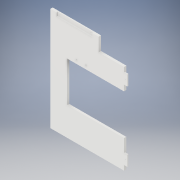
# Autodesk Inventor part: TC001b
Saved by Autodesk Inventor 2017 SP1 (Build 210196100, 196)
## iProperties
Created: 2018-01-07
Part Number: TC001b
Material: ABS Plastic
Document SubType Name: Modeling
Designer: Zach
Density: 1.06 g/cm^3
Appearance: CR White
Author: Zach
Autodesk Inventor part; units mm, degrees
ref_plane "YZ Plane" through (0, 0, 0) normal (1, 0, 0) x (0, 1, 0)
ref_plane "XZ Plane" through (0, 0, 0) normal (0, 1, 0) x (-1, 0, 0)
ref_plane "XY Plane" through (0, 0, 0) normal (0, 0, 1) x (1, 0, 0)
sketch "Sketch1" plane through (0, 0, 0) normal (0, 0, 1) x (1, 0, 0)
  line L0 (0, 0) -> (620, 0)
  line L1 (620, 0) -> (620, 620)
  line L2 (620, 620) -> (0, 620)
  line L3 (0, 620) -> (0, 0)
  line L4 (203.5, 491) -> (416.5, 491)
  line L5 (416.5, 491) -> (416.5, 378)
  line L6 (416.5, 378) -> (203.5, 378)
  line L7 (203.5, 378) -> (203.5, 491)
  point P0 (310, 491)
  point P1 (310, 620)
  dimension "d0" = 620
  dimension "d1" = 620
  dimension "d2" = 213
  dimension "d3" = 113
  dimension "d4" = 129
  constraints: 16 end point, 4 parallel, 2 horizontal, 2 midpoint, 2 perpendicular, 1 vertical alignment
  measures "d0" distance of L2.end L1.end
  measures "d1" distance of L1.end L0.end
  measures "d2" distance of L5.end L6.end
  measures "d3" distance of L4.end L5.end
  measures "d4" distance between parallel lines of L2 L4
extrude "Extrusion1" add sketch "Sketch1" along normal blind 10
sketch "Sketch2" plane through (0, 0, 10) normal (0, 0, 1) x (1, 0, 0)
  line L0 (0, 0) -> (310, 0)
  line L1 (310, 0) -> (310, 435)
  line L2 (310, 435) -> (0, 435)
  line L3 (0, 435) -> (0, 0)
  line L4 (620, 620) -> (0, 620) projected
  line L5 (0, 435) -> (620, 435)
  line L6 (620, 435) -> (620, 620)
  line L7 (620, 620) -> (0, 620)
  line L8 (0, 620) -> (0, 435)
  line L9 (310, 435) -> (620, 435)
  line L10 (620, 435) -> (620, 0)
  line L11 (620, 0) -> (310, 0)
  line L12 (310, 0) -> (310, 435)
  point P0 (310, 620)
  dimension "d7" = 435
  constraints: 24 end point, 6 parallel, 3 horizontal, 3 perpendicular, 1 midpoint, 1 vertical alignment
  measures "d7" distance of L1.end L0.end
extrude "Extrusion2" cut sketch "Sketch2" against normal through all contours L1 L5 L10 L11 | L8 L4 L6 L5 L2
sketch "Sketch3" plane through (0, 0, 10) normal (0, 0, 1) x (1, 0, 0)
  line L0 (310, 0) -> (310, 378) projected
  line L1 (310, 357.5) -> (324, 357.5)
  line L2 (324, 357.5) -> (324, 313.5)
  line L3 (324, 313.5) -> (310, 313.5)
  line L4 (310, 313.5) -> (310, 357.5)
  circle A0 centre (317.5, 335.5) radius 2.5
  line L5 (203.5, 378) -> (310, 378) projected
  line L6 (310, 20.5) -> (324, 20.5)
  line L7 (324, 20.5) -> (324, 64.5)
  line L8 (324, 64.5) -> (310, 64.5)
  line L9 (310, 64.5) -> (310, 20.5)
  circle A1 centre (317.5, 42.5) radius 2.5
  line L10 (0, 0) -> (310, 0) projected
  dimension "d32" = 14
  dimension "d33" = 44
  dimension "d34" = 5
  dimension "d35" = 7.5
  dimension "d36" = 22
  dimension "d37" = 20.5
  dimension "d38" = 14
  dimension "d39" = 44
  dimension "d40" = 5
  dimension "d41" = 7.5
  dimension "d42" = 20.5
  dimension "d43" = 22
  constraints: 16 end point, 4 parallel, 2 centre point, 2 horizontal, 2 perpendicular, 2 point on line
  measures "d32" distance of L2.end L3.end
  measures "d33" distance of L1.end L2.end
  measures "d34" diameter of A0
  measures "d35" distance from line of L0 A0.centre
  measures "d36" distance from line of L1 A0.centre
  measures "d37" distance between parallel lines of L5 L1
  measures "d38" distance of L8.end L7.end
  measures "d39" distance of L7.end L6.end
  measures "d40" diameter of A1
  measures "d41" distance from line of L0 A1.centre
  measures "d42" distance between parallel lines of L10 L6
  measures "d43" distance from line of L6 A1.centre
extrude "Extrusion3" add sketch "Sketch3" against normal blind 5
sketch "Sketch4" plane through (0, 0, 10) normal (0, 0, 1) x (1, 0, 0)
  line L0 (203.5, 435) -> (0, 435) projected
  line L1 (26.75, 435) -> (176.75, 435)
  line L2 (176.75, 435) -> (176.75, 420)
  line L3 (176.75, 420) -> (26.75, 420)
  line L4 (26.75, 420) -> (26.75, 435)
  point P0 (0, 0)
  point P1 (101.75, 435)
  dimension "d18" = 150
  dimension "d19" = 15
  constraints: 8 end point, 2 midpoint, 2 parallel, 1 horizontal, 1 perpendicular, 1 point on line
  measures "d18" distance of L2.end L3.end
  measures "d19" distance of L1.end L2.end
extrude "Extrusion4" cut sketch "Sketch4" against normal blind 5
sketch "Sketch5" plane through (0, 0, 5) normal (0, 0, 1) x (1, 0, 0)
  circle A0 centre (36.75, 427.5) radius 2.5
  circle A1 centre (166.75, 427.5) radius 2.5
  line L0 (26.75, 420) -> (26.75, 435) projected
  line L1 (176.75, 435) -> (176.75, 420) projected
  point P0 (0, 0)
  point P1 (26.75, 427.5)
  dimension "d22" = 5
  dimension "d23" = 5
  dimension "d24" = 10
  dimension "d25" = 10
  constraints: 2 centre point, 2 horizontal alignment, 1 midpoint
  measures "d22" diameter of A0
  measures "d23" diameter of A1
  measures "d24" distance from line of L0 A0.centre
  measures "d25" distance from line of L1 A1.centre
extrude "Extrusion5" cut sketch "Sketch5" against normal through all
sketch "Sketch6" plane through (0, 0, 0) normal (0, 0, -1) x (-1, 0, 0)
  line L0 (-310, 64.5) -> (-310, 313.5) projected
  line L1 (-310, 289) -> (-70, 289)
  line L2 (-70, 289) -> (-70, 119)
  line L3 (-70, 119) -> (-310, 119)
  line L4 (-310, 119) -> (-310, 289)
  line L5 (-310, 313.5) -> (-324, 313.5) projected
  point P0 (0, 0)
  dimension "d44" = 240
  dimension "d45" = 170
  dimension "d55" = 24.5
  constraints: 8 end point, 2 parallel, 1 horizontal, 1 perpendicular, 1 point on line
  measures "d44" distance of L2.end L3.end
  measures "d45" distance of L1.end L2.end
  measures "d55" distance between parallel lines of L5 L1
extrude "Extrusion6" cut sketch "Sketch6" against normal through all
sketch "Sketch7" plane through (0, 0, 0) normal (0, 0, -1) x (-1, 0, 0)
  circle A0 centre (-111, 304) radius 2.5
  circle A1 centre (-151, 304) radius 2.5
  line L0 (-70, 289) -> (-70, 119) projected
  line L1 (-310, 289) -> (-70, 289) projected
  point P0 (0, 0)
  dimension "d48" = 5
  dimension "d49" = 5
  dimension "d50" = 40
  dimension "d51" = 41
  dimension "d52" = 15
  constraints: 2 centre point, 1 horizontal alignment
  measures "d48" diameter of A0
  measures "d49" diameter of A1
  measures "d50" distance of A1.centre A0.centre
  measures "d51" distance from line of L0 A0.centre
  measures "d52" distance from line of L1 A0.centre
extrude "Extrusion7" cut sketch "Sketch7" against normal through all
chamfer "Chamfer1" distance 10 angle 5 1 edges at (190, 119, 0) measured on face at (190, 119, 0.5)
body "Solid1"
